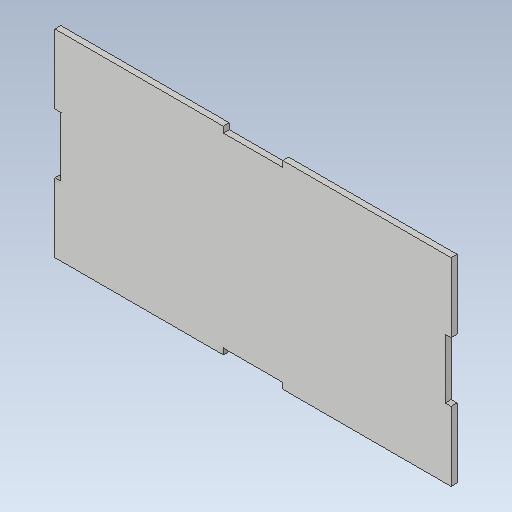
# Autodesk Inventor part: Part1
Saved by Autodesk Inventor 2020 (Build 240168000, 168)
## iProperties
Created: 2020-03-09
Part Number: Part1
Material: Generic
Document SubType Name: Modeling
Designer: tor16003
Density: 1 g/cm^3
Appearance: Default
Author: tor16003
Autodesk Inventor part; units mm, degrees
ref_plane "YZ Plane" through (0, 0, 0) normal (1, 0, 0) x (0, 1, 0)
ref_plane "XZ Plane" through (0, 0, 0) normal (0, 1, 0) x (-1, 0, 0)
ref_plane "XY Plane" through (0, 0, 0) normal (0, 0, 1) x (1, 0, 0)
sketch "Sketch1" plane through (0, 0, 0) normal (0, 0, 1) x (1, 0, 0)
  line L0 (0, 0) -> (85, 0)
  line L1 (85, 0) -> (85, 3)
  line L2 (85, 3) -> (115, 3)
  line L3 (115, 3) -> (115, 0)
  line L4 (200, 0) -> (115, 0)
  line L5 (0, 100) -> (85, 100)
  line L6 (85, 100) -> (85, 97)
  line L7 (85, 97) -> (115, 97)
  line L8 (115, 97) -> (115, 100)
  line L9 (115, 100) -> (200, 100)
  line L10 (0, 100) -> (0, 65)
  line L11 (0, 65) -> (3, 65)
  line L12 (3, 65) -> (3, 35)
  line L13 (3, 35) -> (0, 35)
  line L14 (0, 35) -> (0, 0)
  line L15 (200, 100) -> (200, 65)
  line L16 (200, 65) -> (197, 65)
  line L17 (197, 65) -> (197, 35)
  line L18 (197, 35) -> (200, 35)
  line L19 (200, 35) -> (200, 0)
  dimension "d1" = 200
  dimension "d9" = 85
  dimension "d10" = 85
  dimension "d12" = 3
  dimension "d13" = 100
  dimension "d14" = 3
  dimension "d15" = 35
  dimension "d16" = 35
  dimension "d17" = 3
  constraints: 40 end point, 14 perpendicular, 5 collinear, 3 equal length, 3 horizontal, 3 point on line, 3 vertical
  measures "d1" distance of L9.end L5.start
  measures "d9" distance of L0.start L0.end
  measures "d10" distance of L4.start L3.end
  measures "d12" distance of L5.end L6.end
  measures "d13" distance of L4.start L9.end
  measures "d14" distance of L0.end L1.end
  measures "d15" distance of L13.end L0.start
  measures "d16" distance of L5.start L10.end
  measures "d17" distance of L10.end L11.end
extrude "Extrusion1" add sketch "Sketch1" along normal blind 3
body "Solid1"
